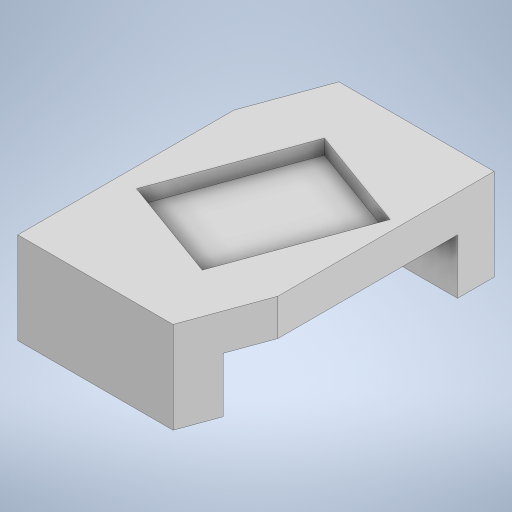
# Autodesk Inventor part: base_obj3
Saved by Autodesk Inventor 2023.2 (Build 272271030, 271C)
## iProperties
Created: 2023-02-25
Part Number: base_obj3
Material: Generic
Document SubType Name: Modeling
Designer: Cris Pat
Density: 1 g/cm^3
Appearance: Default
Author: Cris Pat
Autodesk Inventor part; units mm, degrees
ref_plane "XY Plane" through (0, 0, 0) normal (0, 0, 1) x (1, 0, 0)
sketch "Sketch1" plane through (0, 0, 0) normal (0, 1, 0) x (-1, 0, 0)
  line L0 (-25, -40) -> (25, -40) construction
  line L1 (25, -40) -> (25, 40) construction
  line L2 (25, 40) -> (-25, 40) construction
  line L3 (-25, 40) -> (-25, -40) construction
  line L4 (-25, 19) -> (-17.3566, 40)
  line L5 (17.3566, -40) -> (25, -19)
  line L6 (25, -19) -> (25, 40)
  line L7 (25, 40) -> (-17.3566, 40)
  line L8 (-25, 19) -> (-25, -40)
  line L9 (-25, -40) -> (17.3566, -40)
  point P0 (0, 0)
  point P1 (25, 0)
  point P2 (0, -40)
  dimension "d0" = 50
  dimension "d1" = 80
  dimension "d2" = 21
  dimension "d3" = 20
  dimension "d4" = 20
  dimension "d5" = 21
  constraints: 20 end point, 3 perpendicular, 3 vertical alignment, 2 midpoint, 2 parallel, 2 point on line, 1 collinear, 1 horizontal, 1 horizontal alignment, 1 vertical
  measures "d0" distance of L2.end L1.end
  measures "d1" distance of L1.end L0.end
  measures "d2" distance of L4.start L2.end
  measures "d3" angle of L3 L4
  measures "d4" angle of L1 L5
  measures "d5" distance of L0.end L5.end
extrude "Extrusion1" add sketch "Sketch1" along normal blind 25
ref_plane "Work Plane1" through (25.25, 0, 0) normal (1, 0, 0) x (0, 1, 0)
sketch "Sketch2" plane through (25.25, 0, 0) normal (1, 0, 0) x (0, 1, 0)
  line L0 (0, 40) -> (0, 19) construction
  line L1 (0, 19) -> (25, 19) construction
  line L2 (25, 40) -> (25, 19) construction
  line L3 (0, 40) -> (25, 40) construction
  line L4 (0, 19) -> (0, -40) construction
  line L5 (0, -40) -> (25, -40) construction
  line L6 (25, 19) -> (25, -40) construction
  line L7 (0, 19) -> (25, 19) construction
  line L8 (0, 30) -> (0, -30)
  line L9 (0, 30) -> (15, 30)
  line L10 (15, 30) -> (15, -30)
  line L11 (15, -30) -> (0, -30)
  point P0 (0, 0)
  dimension "d9" = 60
  dimension "d10" = 10
  dimension "d11" = 15
  constraints: 8 end point, 2 vertical, 1 horizontal, 1 perpendicular, 1 vertical alignment
  measures "d9" distance of L8.start L8.end
  measures "d10" distance of L0.start L8.start
  measures "d11" distance of L8.start L9.end
extrude "Extrusion2" cut sketch "Sketch2" against normal through all
ref_plane "Work Plane2" through (0, 25, 0) normal (0, 1, 0) x (-1, 0, 0)
sketch "Sketch3" plane through (0, 25, 0) normal (0, 1, 0) x (-1, 0, 0)
  line L0 (17.3566, -40) -> (25, -19) construction
  line L1 (25, -19) -> (25, 40) construction
  line L2 (25, 40) -> (-17.3566, 40) construction
  line L3 (-17.3566, 40) -> (-25, 19) construction
  line L4 (-25, 19) -> (-25, -40) construction
  line L5 (-25, -40) -> (17.3566, -40) construction
  line L6 (6.0192, -24.6856) -> (-22.1716, -14.425)
  line L7 (-22.1716, -14.425) -> (-8.4908, 23.1627)
  line L8 (-8.4908, 23.1627) -> (19.7, 12.9021)
  line L9 (19.7, 12.9021) -> (6.0192, -24.6856)
  point P0 (0, 0)
  dimension "d15" = 30
  dimension "d16" = 40
  dimension "d17" = 30
  dimension "d18" = 25
  dimension "d19" = 70
  dimension "d20" = 5.3
  constraints: 8 end point, 2 perpendicular
  measures "d15" distance of L6.start L6.end
  measures "d16" distance of L6.end L7.end
  measures "d17" distance of L7.end L8.end
  measures "d18" distance from line of L4.end L6
  measures "d19" angle of L4 L6
  measures "d20" horizontal distance of L1.end L8.end
extrude "Extrusion3" cut sketch "Sketch3" against normal blind 4
body "Solid1"
